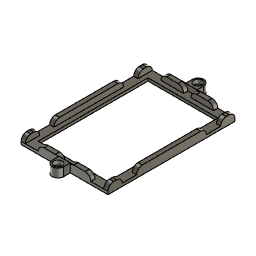
base_para_proto_chica (Autodesk Fusion 360 design; units mm, degrees)
Autodesk Fusion 360 part; units mm, degrees
sketch "Sketch4" plane through (0, 0, 0) normal (0, 0, 1) x (1, 0, 0)
  line L0 (0, 0) -> (54.8, 0)
  line L1 (54.8, 0) -> (54.8, 82.8)
  line L2 (54.8, 82.8) -> (0, 82.8)
  line L3 (0, 82.8) -> (0, 0)
  line L4 (57.8, -3) -> (57.8, 85.8)
  line L5 (-3, 85.8) -> (-3, -3)
  line L6 (0, 41.4) -> (54.8, 41.4) construction
  line L7 (27.4, 0) -> (27.4, 1.8094) construction
  line L8 (27.4, 1.8094) -> (27.4, 82.8) construction
  line L9 (23.4, 85.8) -> (23.4, 90.4)
  line L10 (31.4, 90.4) -> (31.4, 85.8)
  line L11 (23.4, -3) -> (23.4, -7.6)
  line L12 (31.4, -7.6) -> (31.4, -3)
  arc A0 (31.4, 90.4) -> (23.4, 90.4) centre (27.4, 90.4) ccw
  arc A1 (23.4, -7.6) -> (31.4, -7.6) centre (27.4, -7.6) ccw
  line L13 (-3, -3) -> (23.4, -3)
  line L14 (31.4, -3) -> (57.8, -3)
  line L15 (57.8, 85.8) -> (31.4, 85.8)
  line L16 (23.4, 85.8) -> (-3, 85.8)
  line L17 (3, 3) -> (51.8, 3)
  line L18 (51.8, 3) -> (51.8, 79.8)
  line L19 (51.8, 79.8) -> (3, 79.8)
  line L20 (3, 79.8) -> (3, 3)
  point P0 (27.4, 90.4)
  point P1 (27.4, -7.6)
  dimension "d22" = 54.8
  dimension "d23" = 82.8
  dimension "d25" = 8
  dimension "d26" = 49
  dimension "d27" = 49
  dimension "d30" = -3
  constraint horizontal L0
  constraint vertical L1
  constraint horizontal L2
  constraint vertical L3
  constraint coincident L0.start L3.end
  constraint midpoint L3 L6.start
  constraint midpoint L1 L6.end
  constraint midpoint L0 L7.start
  constraint perpendicular L0 L7
  constraint midpoint L2 L8.end
  constraint perpendicular L2 L8
  constraint equal A0 A1
  constraint parallel L9 L10
  constraint coincident P0 A0.centre
  constraint parallel L11 L12
  constraint coincident L12.end L13
  constraint coincident P1 A1.centre
  constraint parallel L0 L13
  constraint parallel L1 L4
  constraint parallel L2 L15
  constraint parallel L3 L5
  constraint collinear L13 L14
  constraint collinear L15 L16
  measures "d22" distance of L0.start L0.end
  measures "d23" distance of L0.start L2.end
  measures "d25" diameter of A0
  measures "d26" distance of P0 L6
  measures "d27" distance of P1 L6
extrude "Extrude5" add sketch "Sketch4" along normal blind 2 contours L0 L1 L2 L3
extrude "Extrude6" add sketch "Sketch4" along normal blind 6 contours L4 L5 L9 L10 L11 L12 A0 A1 L13 L14 L15 L16
sketch "Sketch5" plane through (0, 0, 6) normal (0, 0, 1) x (-1, 0, 0)
  line L0 (0, 0) -> (0, -82.8)
  line L1 (0, -82.8) -> (-54.8, -82.8)
  line L2 (-54.8, -82.8) -> (-54.8, 0)
  line L3 (-54.8, 0) -> (0, 0)
  arc A0 (-31.4, -90.4) -> (-23.4, -90.4) centre (-27.4, -90.4) ccw
  line L4 (-23.4, -90.4) -> (-23.4, -85.8)
  line L5 (-23.4, -85.8) -> (3, -85.8)
  line L6 (3, -85.8) -> (3, 3)
  line L7 (3, 3) -> (-23.4, 3)
  line L8 (-23.4, 3) -> (-23.4, 7.6)
  arc A1 (-23.4, 7.6) -> (-31.4, 7.6) centre (-27.4, 7.6) ccw
  line L9 (-31.4, 7.6) -> (-31.4, 3)
  line L10 (-31.4, 3) -> (-57.8, 3)
  line L11 (-57.8, 3) -> (-57.8, -85.8)
  line L12 (-57.8, -85.8) -> (-31.4, -85.8)
  line L13 (-31.4, -85.8) -> (-31.4, -90.4)
  circle A2 centre (-27.4, -90.4) radius 3
  circle A3 centre (-27.4, 7.6) radius 3
  dimension "d35" = 6
  constraint concentric A0 A2
  constraint concentric A1 A3
  constraint equal A2 A3
  measures "d35" diameter of A2
extrude "Extrude7" cut sketch "Sketch5" against normal blind 3 contours A2 | A3
sketch "Sketch6" plane through (0, 0, 3) normal (0, 0, 1) x (-1, 0, 0)
  circle A0 centre (-27.4, -90.4) radius 3
  circle A1 centre (-27.4, -90.4) radius 1.6
  circle A2 centre (-27.4, 7.6) radius 1.6
  dimension "d38" = 3.2
  dimension "d39" = 3.2
  constraint concentric A0 A1
  measures "d38" diameter of A1
  measures "d39" diameter of A2
extrude "Extrude8" cut sketch "Sketch6" against normal blind 4 contours A1 | A2
sketch "Sketch7" plane through (0, 0, 6) normal (0, 0, 1) x (-1, 0, 0)
  circle A0 centre (-27.4, -90.4) radius 3
  circle A1 centre (-27.4, 7.6) radius 3
  line L0 (0, 0) -> (0, -82.8)
  line L1 (0, -82.8) -> (-54.8, -82.8)
  line L2 (-54.8, -82.8) -> (-54.8, 0)
  line L3 (-54.8, 0) -> (0, 0)
  arc A2 (-31.4, -90.4) -> (-23.4, -90.4) centre (-27.4, -90.4) ccw
  line L4 (-23.4, -90.4) -> (-23.4, -85.8)
  line L5 (-23.4, -85.8) -> (3, -85.8)
  line L6 (3, -85.8) -> (3, 3)
  line L7 (3, 3) -> (-23.4, 3)
  line L8 (-23.4, 3) -> (-23.4, 7.6)
  arc A3 (-23.4, 7.6) -> (-31.4, 7.6) centre (-27.4, 7.6) ccw
  line L9 (-31.4, 7.6) -> (-31.4, 3)
  line L10 (-31.4, 3) -> (-57.8, 3)
  line L11 (-57.8, 3) -> (-57.8, -85.8)
  line L12 (-57.8, -85.8) -> (-31.4, -85.8)
  line L13 (-31.4, -85.8) -> (-31.4, -90.4)
  line L14 (4.5, -17) -> (-1.5, -17)
  line L15 (-1.5, -17) -> (-1.5, -7)
  line L16 (-1.5, -7) -> (4.5, -7)
  line L17 (4.5, -7) -> (4.5, -17)
  line L18 (4.5, -17) -> (-1.5, -7) construction
  line L19 (-1.5, -17) -> (4.5, -7) construction
  line L20 (3, -41.4) -> (-57.8, -41.4) construction
  line L21 (-27.4, 0) -> (-27.4, -82.8) construction
  line L22 (-1.5, -75.8) -> (4.5, -75.8)
  line L23 (4.5, -75.8) -> (4.5, -65.8)
  line L24 (-1.5, -65.8) -> (-1.5, -75.8)
  line L25 (4.5, -65.8) -> (-1.5, -65.8)
  line L26 (0, 0) -> (-9, 0)
  line L27 (-9, 0) -> (-9, 3)
  line L28 (-9, 3) -> (0, 3)
  line L29 (0, 3) -> (0, 0)
  line L30 (-54.8, 0) -> (-45.8, 0)
  line L31 (-45.8, 3) -> (-54.8, 3)
  line L32 (-54.8, 3) -> (-54.8, 0)
  line L33 (-45.8, 0) -> (-45.8, 3)
  line L34 (-29.9523, 2.9079) -> (-24.9523, 2.9079)
  line L35 (-24.9523, 2.9079) -> (-24.9523, -0.0921)
  line L36 (-24.9523, -0.0921) -> (-29.9523, -0.0921)
  line L37 (-29.9523, -0.0921) -> (-29.9523, 2.9079)
  line L38 (-29.9523, 2.9079) -> (-24.9523, -0.0921) construction
  line L39 (-24.9523, 2.9079) -> (-29.9523, -0.0921) construction
  line L40 (-24.9523, -82.7079) -> (-29.9523, -82.7079)
  line L41 (-24.9523, -85.7079) -> (-24.9523, -82.7079)
  line L42 (-29.9523, -85.7079) -> (-24.9523, -85.7079)
  line L43 (-29.9523, -82.7079) -> (-29.9523, -85.7079)
  line L44 (0, -82.8) -> (-9, -82.8)
  line L45 (-9, -82.8) -> (-9, -85.8)
  line L46 (-9, -85.8) -> (0, -85.8)
  line L47 (0, -85.8) -> (0, -82.8)
  line L48 (-45.8, -82.8) -> (-45.8, -85.8)
  line L49 (-45.8, -85.8) -> (-54.8, -85.8)
  line L50 (-54.8, -85.8) -> (-54.8, -82.8)
  line L51 (-54.8, -82.8) -> (-45.8, -82.8)
  line L52 (-59.3, -65.8) -> (-53.3, -65.8)
  line L53 (-53.3, -65.8) -> (-53.3, -75.8)
  line L54 (-53.3, -75.8) -> (-59.3, -75.8)
  line L55 (-59.3, -75.8) -> (-59.3, -65.8)
  line L56 (-53.3, -17) -> (-53.3, -7)
  line L57 (-53.3, -7) -> (-59.3, -7)
  line L58 (-59.3, -7) -> (-59.3, -17)
  line L59 (-59.3, -17) -> (-53.3, -17)
  point P0 (1.5, -12)
  point P1 (-27.4523, 1.4079)
  dimension "d42" = 10
  dimension "d43" = 12
  dimension "d44" = 9
  dimension "d45" = 5
  dimension "d46" = 3
  constraint horizontal L14
  constraint perpendicular L14 L15
  constraint parallel L14 L16
  constraint parallel L15 L17
  constraint coincident L18 P0
  constraint coincident L19 P0
  constraint midpoint L6 L20.start
  constraint midpoint L11 L20.end
  constraint midpoint L3 L21.start
  constraint midpoint L1 L21.end
  constraint symmetric L14.start L20 L23.end
  constraint symmetric L14.end L20 L24.start
  constraint symmetric L15.end L20 L22.start
  constraint symmetric L16.end L20 L22.end
  constraint horizontal L26
  constraint vertical L27
  constraint horizontal L28
  constraint vertical L29
  constraint coincident L0.start L3.end
  constraint symmetric L21 L0.start L2.end
  constraint symmetric L21 L26.end L30.end
  constraint symmetric L21 L27.end L31.start
  constraint symmetric L21 L28.end L31.end
  constraint horizontal L34
  constraint perpendicular L34 L35
  constraint parallel L34 L36
  constraint parallel L35 L37
  constraint coincident L38 P1
  constraint coincident L39 P1
  constraint symmetric L20 L34.start L42.start
  constraint symmetric L20 L34.end L41.start
  constraint symmetric L20 L35.end L40.start
  constraint symmetric L20 L36.end L40.end
  constraint symmetric L20 L0.start L0.end
  constraint symmetric L20 L26.end L44.end
  constraint symmetric L20 L27.end L45.end
  constraint symmetric L20 L28.end L46.end
  constraint symmetric L20 L2.end L1.end
  constraint symmetric L20 L30.end L48.start
  constraint symmetric L20 L31.start L48.end
  constraint symmetric L20 L31.end L49.end
  constraint symmetric L14.start L21 L58.end
  constraint symmetric L14.end L21 L56.start
  constraint symmetric L15.end L21 L56.end
  constraint symmetric L16.end L21 L57.end
  constraint symmetric L21 L22.start L53.end
  constraint symmetric L21 L22.end L54.end
  constraint symmetric L21 L23.end L52.start
  constraint symmetric L21 L24.start L52.end
  measures "d42" distance of L14.end L15.end
  measures "d43" distance of L3 P0
  measures "d44" distance of L0.start L26.end
  measures "d45" distance of L35.end L36.end
  measures "d46" distance of L34.end L35.end
extrude "Extrude9" cut sketch "Sketch7" against normal blind 4 contours L3 L7 L26 L27 L28 L29 | L0 L6 L14 L16 | L0 L14 L15 L16 | L6 L14 L16 L17 | L3 L34 L35 L37 | L0 L6 L22 L25 | L0 L22 L24 L25 | L6 L22 L23 L25 | L3 L10 L30 L31 L32 L33 | L1 L5 L44 L45 L46 L47 | L2 L56 L57 L59 | L2 L11 L57 L59 | L1 L41 L42 L43 | L11 L57 L58 L59 | L2 L52 L53 L54 | L2 L11 L52 L54 | L1 L12 L48 L49 L50 L51 | L11 L52 L54 L55
fillet "Empalme4" radius 4 20 edges at (56.3, 17, 6) (56.3, 7, 6) (56.3, -3, 6) (45.8, -1.5, 6) (29.9523, -1.454, 6) (24.9523, -1.454, 6) (9, -1.5, 6) (-1.5, -3, 6) (-1.5, 7, 6) (-1.5, 17, 6) (56.3, 65.8, 6) (56.3, 75.8, 6) (56.3, 85.8, 6) (45.8, 84.3, 6) (29.9523, 84.254, 6) (24.9523, 84.254, 6) (-1.5, 75.8, 6) (-1.5, 65.8, 6) (-1.5, 85.8, 6) (9, 84.3, 6)
